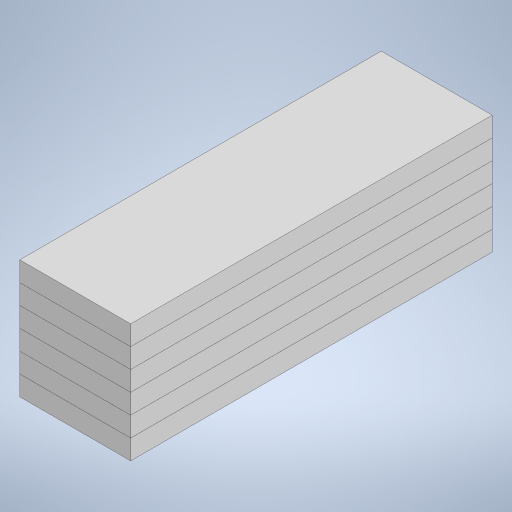
# Autodesk Inventor part: Battery_model
Saved by Autodesk Inventor 2024 (Build 280153000, 153)
## iProperties
Created: 2024-03-13
Part Number: Battery_model
Material: Generic
Document SubType Name: Modeling
Designer: nicoe
Density: 1 g/cm^3
Appearance: Default
Author: nicoe
Autodesk Inventor part; units mm, degrees
ref_plane "YZ Plane" through (0, 0, 0) normal (1, 0, 0) x (0, 1, 0)
ref_plane "XZ Plane" through (0, 0, 0) normal (0, 1, 0) x (-1, 0, 0)
ref_plane "XY Plane" through (0, 0, 0) normal (0, 0, 1) x (1, 0, 0)
sketch "Sketch1" plane through (0, 0, 0) normal (0, 1, 0) x (-1, 0, 0)
  line L0 (21, 68.5) -> (-21, 68.5)
  line L1 (-21, 68.5) -> (-21, -68.5)
  line L2 (-21, -68.5) -> (21, -68.5)
  line L3 (21, -68.5) -> (21, 68.5)
  point P0 (0, 0)
  dimension "d0" = 42
  dimension "d1" = 137
  dimension "d2" = 21
  dimension "d3" = 68.5
  constraints: 8 end point, 2 parallel, 1 horizontal, 1 perpendicular
  measures "d0" distance of L2.end L1.end
  measures "d1" distance of L1.end L0.end
  measures "d2" distance from line of point (0, 0) L3
  measures "d3" distance from line of point (0, 0) L2
extrude "Extrusion1" add sketch "Sketch1" along normal blind 7.5
sketch "Sketch3" plane through (0, 7.5, 0) normal (0, 1, 0) x (1, 0, 0)
  line L0 (21, -68.5) -> (21, 68.5) projected
  line L1 (21, 68.5) -> (-21, 68.5) projected
  line L2 (-21, 68.5) -> (-21, -68.5) projected
  line L3 (-21, -68.5) -> (21, -68.5) projected
  line L4 (-20.99, -68.49) -> (-20.99, 68.49)
  line L5 (-20.99, 68.49) -> (20.99, 68.49)
  line L6 (20.99, 68.49) -> (20.99, -68.49)
  line L7 (20.99, -68.49) -> (-20.99, -68.49)
  point P0 (0, 0)
  dimension "d6" = 0.01
  constraints: 8 end point, 3 other
  measures "d6" distance between parallel lines of L2 L4
extrude "Extrusion2" add sketch "Sketch3" along normal blind 7.5 contours L4 L5 L6 L7
sketch "Sketch4" plane through (0, 15, 0) normal (0, 1, 0) x (1, 0, 0)
  line L0 (20.99, -68.49) -> (-20.99, -68.49) projected
  line L1 (-20.99, -68.49) -> (-20.99, 68.49) projected
  line L2 (-20.99, 68.49) -> (20.99, 68.49) projected
  line L3 (20.99, 68.49) -> (20.99, -68.49) projected
  line L4 (21, -68.5) -> (21, 68.5) projected
  line L5 (21, 68.5) -> (-21, 68.5) projected
  line L6 (-21, 68.5) -> (-21, -68.5) projected
  line L7 (-21, -68.5) -> (21, -68.5) projected
  point P0 (0, 0)
extrude "Extrusion3" add sketch "Sketch4" along normal blind 7.5 contours L0 L1 L2 L3 | L7 L6 L5 L4
sketch "Sketch5" plane through (0, 22.5, 0) normal (0, 1, 0) x (1, 0, 0)
  line L0 (21, 68.5) -> (-21, 68.5) projected
  line L1 (-21, 68.5) -> (-21, -68.5) projected
  line L2 (-21, -68.5) -> (21, -68.5) projected
  line L3 (21, -68.5) -> (21, 68.5) projected
  line L4 (-20.99, -68.49) -> (-20.99, 68.49)
  line L5 (-20.99, 68.49) -> (20.99, 68.49)
  line L6 (20.99, 68.49) -> (20.99, -68.49)
  line L7 (20.99, -68.49) -> (-20.99, -68.49)
  point P0 (0, 0)
  dimension "d11" = 0.01
  constraints: 8 end point, 3 other
  measures "d11" distance between parallel lines of L1 L4
extrude "Extrusion4" add sketch "Sketch5" along normal blind 7.5 contours L4 L5 L6 L7
sketch "Sketch6" plane through (0, 30, 0) normal (0, 1, 0) x (1, 0, 0)
  line L0 (20.99, -68.49) -> (-20.99, -68.49) projected
  line L1 (-20.99, -68.49) -> (-20.99, 68.49) projected
  line L2 (-20.99, 68.49) -> (20.99, 68.49) projected
  line L3 (20.99, 68.49) -> (20.99, -68.49) projected
  line L4 (21, 68.5) -> (-21, 68.5) projected
  line L5 (-21, 68.5) -> (-21, -68.5) projected
  line L6 (-21, -68.5) -> (21, -68.5) projected
  line L7 (21, -68.5) -> (21, 68.5) projected
  point P0 (0, 0)
extrude "Extrusion5" add sketch "Sketch6" along normal blind 7.5 contours L0 L1 L2 L3 | L7 L6 L5 L4
sketch "Sketch7" plane through (0, 37.5, 0) normal (0, 1, 0) x (1, 0, 0)
  line L0 (-21, 68.5) -> (-21, -68.5) projected
  line L1 (-21, -68.5) -> (21, -68.5) projected
  line L2 (21, -68.5) -> (21, 68.5) projected
  line L3 (21, 68.5) -> (-21, 68.5) projected
  line L4 (-21.01, -68.51) -> (-21.01, 68.51)
  line L5 (-21.01, 68.51) -> (21.01, 68.51)
  line L6 (21.01, 68.51) -> (21.01, -68.51)
  line L7 (21.01, -68.51) -> (-21.01, -68.51)
  point P0 (0, 0)
  dimension "d16" = 0.01
  constraints: 8 end point, 3 other
  measures "d16" distance between parallel lines of L0 L4
extrude "Extrusion6" add sketch "Sketch7" along normal blind 7.5 contours L3 L2 L1 L0 | L4 L5 L6 L7
equation "\"d2\" = 0.5 * d0"
equation "\"d3\" = 0.5 * d1"
body "Solid1"
